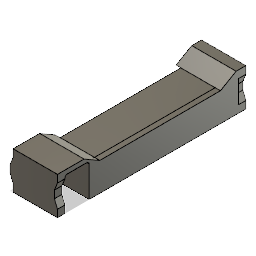
Key v4 (Autodesk Fusion 360 design; units mm, degrees)
Autodesk Fusion 360 part; units mm, degrees
sketch "Sketch1" plane through (0, 0, 0) normal (0, 1, 0) x (1, 0, 0)
  line L0 (14.75, 62.5) -> (-14.75, 62.5)
  line L1 (-14.75, 62.5) -> (-14.75, -62.5)
  line L2 (-14.75, -62.5) -> (14.75, -62.5)
  line L3 (14.75, -62.5) -> (14.75, 62.5)
  line L4 (14.75, 62.5) -> (-14.75, -62.5) construction
  line L5 (-14.75, 62.5) -> (14.75, -62.5) construction
  dimension "d1" = 29.5
  dimension "d4" = 125
extrude "Extrude1" add sketch "Sketch1" along normal blind 25
sketch "Sketch2" plane through (14.75, 0, 0) normal (1, 0, 0) x (0, 0, -1)
  line L0 (-62.5, 0) -> (62.5, 0)
  line L1 (62.5, 25) -> (-62.5, 25)
  line L2 (-62.5, 25) -> (-62.5, 0)
  line L3 (-57.5, 0) -> (-41.5, 0)
  line L4 (-41.5, 0) -> (-41.5, 22)
  line L5 (-41.5, 22) -> (-57.5, 22)
  line L6 (-57.5, 22) -> (-57.5, 0)
  dimension "d5" = 16
  dimension "d6" = 5
  dimension "d70" = 3
  measures "d6" distance of L2 L6
  measures "d70" distance of L1 L5
extrude "Extrude2" cut sketch "Sketch2" against normal through all
sketch "Sketch3" plane through (-14.75, 0, 0) normal (-1, 0, 0) x (0, 0, 1)
  line L0 (57.5, 22) -> (57.5, 0)
  line L1 (57.5, 0) -> (62.5, 0)
  line L2 (62.5, 0) -> (62.5, 25)
  line L3 (62.5, 25) -> (-62.5, 25)
  line L4 (-62.5, 25) -> (-62.5, 0)
  line L5 (-62.5, 0) -> (41.5, 0)
  line L6 (41.5, 0) -> (41.5, 22)
  line L7 (41.5, 22) -> (57.5, 22)
  line L8 (-57.5, 0) -> (37.5, 0)
  line L9 (37.5, 0) -> (37.5, 14.5)
  line L10 (37.5, 14.5) -> (-57.5, 14.5)
  line L11 (-57.5, 14.5) -> (-57.5, 0)
  dimension "d12" = 4
  dimension "d51" = 5
  dimension "d69" = 10.5
  measures "d12" distance of L6 L9
  measures "d51" distance of L4 L11
  measures "d69" distance of L3 L10
extrude "Extrude3" cut sketch "Sketch3" against normal blind 26 contours L5 L8 L9 L10 L11
sketch "Sketch4" plane through (-14.75, 0, 0) normal (-1, 0, 0) x (0, 0, 1)
  line L0 (37.5, 14.5) -> (37.5, 0)
  line L1 (37.5, 0) -> (41.5, 0)
  line L2 (41.5, 0) -> (41.5, 22)
  line L3 (41.5, 22) -> (57.5, 22)
  line L4 (57.5, 22) -> (57.5, 0)
  line L5 (57.5, 0) -> (62.5, 0)
  line L6 (62.5, 0) -> (62.5, 25)
  line L7 (62.5, 25) -> (-62.5, 25)
  line L8 (-62.5, 25) -> (-62.5, 0)
  line L9 (-62.5, 0) -> (-57.5, 0)
  line L10 (-57.5, 14.5) -> (37.5, 14.5)
  line L11 (-55.8923, 25) -> (-45.5, 19)
  line L12 (-45.5, 19) -> (34.5, 19)
  line L13 (34.5, 19) -> (44.8923, 25)
  line L14 (-57.5, 0) -> (-57.5, 14.5)
  dimension "d16" = 6
  dimension "d44" = 150
  dimension "d45" = 150
  dimension "d46" = 80
  dimension "d49" = 28
  measures "d16" distance of origin
  measures "d44" angle of L11 L12
  measures "d45" angle of L12 L13
extrude "Extrude4" cut sketch "Sketch4" against normal through all contours L7 L11 L12 L13
sketch "Sketch5" plane through (-14.75, 0, 0) normal (-1, 0, 0) x (0, 0, 1)
  line L0 (44.8923, 25) -> (34.5, 19)
  line L1 (34.5, 19) -> (-45.5, 19)
  line L2 (-45.5, 19) -> (-55.8923, 25)
  line L3 (-62.5, 25) -> (-62.5, 0)
  line L4 (-62.5, 0) -> (-57.5, 0)
  line L5 (-57.5, 14.5) -> (37.5, 14.5)
  line L6 (37.5, 14.5) -> (37.5, 0)
  line L7 (37.5, 0) -> (41.5, 0)
  line L8 (41.5, 0) -> (41.5, 22)
  line L9 (-50.5, 19) -> (39.5, 19)
  line L10 (39.5, 19) -> (39.5, 15.8)
  line L11 (39.5, 15.8) -> (-50.5, 15.8)
  line L12 (-50.5, 15.8) -> (-50.5, 19)
  line L13 (-57.5, 0) -> (-57.5, 14.5)
  line L14 (41.5, 22) -> (57.5, 22)
  line L15 (57.5, 22) -> (57.5, 0)
  line L16 (57.5, 0) -> (62.5, 0)
  line L17 (62.5, 0) -> (62.5, 25)
  line L18 (-55.8923, 25) -> (-62.5, 25)
  line L19 (62.5, 25) -> (44.8923, 25)
  dimension "d21" = 5
  dimension "d22" = 3.2
  dimension "d48" = 5
  measures "d21" distance of L12
extrude "Extrude5" cut sketch "Sketch5" against normal blind 26 contours L1 L9 L10 L11 L12
ref_plane "WorkPlane1" through (0, 12.5, 0) normal (0, 0, -1) x (-1, 0, 0)
sketch "Sketch6" plane through (0, 0, -62.5) normal (0, 0, -1) x (-1, 0, 0)
  line L0 (-14.75, 0) -> (14.75, 0)
  line L1 (14.75, 0) -> (14.75, 25)
  line L2 (-14.75, 25) -> (-14.75, 0)
  line L3 (14.75, 25) -> (-14.75, 25)
  line L4 (14.75, 20) -> (14.75, 5)
  line L5 (14.75, 5) -> (16.75, 10)
  line L6 (16.75, 10) -> (16.75, 15)
  line L7 (16.75, 15) -> (14.75, 20)
  line L8 (16.75, 12.5) -> (14.75, 12.5) construction
  dimension "d52" = 5
  dimension "d53" = 5
  dimension "d54" = 2
  dimension "d55" = 5
  measures "d52" distance of L0
  measures "d53" distance of L3
  measures "d54" distance of L4 L6
sketch "Sketch7" plane through (0, 0, -62.5) normal (0, 0, -1) x (-1, 0, 0)
  line L0 (14.75, 0) -> (-14.75, 0)
  line L1 (-14.75, 0) -> (-14.75, 25)
  line L2 (-14.75, 20) -> (-14.75, 5)
  line L3 (-14.75, 5) -> (-12.75, 10)
  line L4 (-14.75, 20) -> (-12.75, 15)
  line L5 (-12.75, 15) -> (-12.75, 10)
  line L6 (-12.75, 12.5) -> (-14.75, 12.5) construction
  dimension "d56" = 5
  dimension "d57" = 5
  dimension "d58" = 2
  dimension "d59" = 5
  measures "d58" distance of L2 L5
extrude "Extrude6" add sketch "Sketch6" against normal blind 5 contours L1 L4 L5 L6 L7
extrude "Extrude7" cut sketch "Sketch7" against normal up to surface (5 mm away)
mirror "Mirror1" about plane through (0, 12.5, 0) normal (0, 0, -1) of "Extrude6", "Extrude7"
sketch "Sketch9" plane through (0, 0, 41.5) normal (0, 0, 1) x (1, 0, 0)
  line L0 (-14.75, 22) -> (-14.75, 0)
  line L1 (-14.75, 0) -> (14.75, 0)
  line L2 (14.75, 0) -> (14.75, 22)
  line L3 (1.25, 19.8) -> (-4.75, 19.8)
  line L4 (-4.75, 19.8) -> (-4.75, 13.8)
  line L5 (-4.75, 13.8) -> (1.25, 13.8)
  line L6 (1.25, 13.8) -> (1.25, 19.8)
  line L7 (1.25, 19.8) -> (-4.75, 13.8) construction
  line L8 (-4.75, 19.8) -> (1.25, 13.8) construction
  line L9 (-14.75, 15.8) -> (11.25, 15.8) construction
  line L10 (-1.75, 15.8) -> (-1.75, 16.8) construction
  line L11 (14.75, 22) -> (-14.75, 22)
  dimension "d39" = 6
  dimension "d67" = 4
  measures "d67" distance of L3 L9
extrude "Extrude9" cut sketch "Sketch9" against normal blind 2 contours L3 L4 L5 L6
sketch "Sketch10" plane through (0, 0, -62.5) normal (0, 0, -1) x (-1, 0, 0)
  line L0 (-12.75, 10) -> (-14.75, 5)
  line L1 (-14.75, 5) -> (-14.75, 0)
  line L2 (-14.75, 0) -> (14.75, 0)
  line L3 (14.75, 0) -> (14.75, 5)
  line L4 (14.75, 5) -> (16.75, 10)
  line L5 (16.75, 10) -> (16.75, 15)
  line L6 (16.75, 15) -> (14.75, 20)
  line L7 (14.75, 20) -> (14.75, 25)
  line L8 (14.75, 25) -> (-14.75, 25)
  line L9 (-14.75, 25) -> (-14.75, 20)
  line L10 (-14.75, 20) -> (-12.75, 15)
  line L11 (-12.75, 15) -> (-12.75, 10)
  circle A0 centre (1.75, 8) radius 2
  line L12 (14.75, 14.5) -> (-11.25, 14.5)
  line L13 (1.75, 8) -> (1.75, 14.5) construction
  dimension "d60" = 4
  dimension "d61" = 8
  measures "d60" diameter of A0
  measures "d61" distance of L2
extrude "Extrude10" cut sketch "Sketch10" against normal blind 5 contours A0
fillet "Fillet3" radius 1.5 2 edges at (0, 22, 41.5) (0, 22, 57.5)
